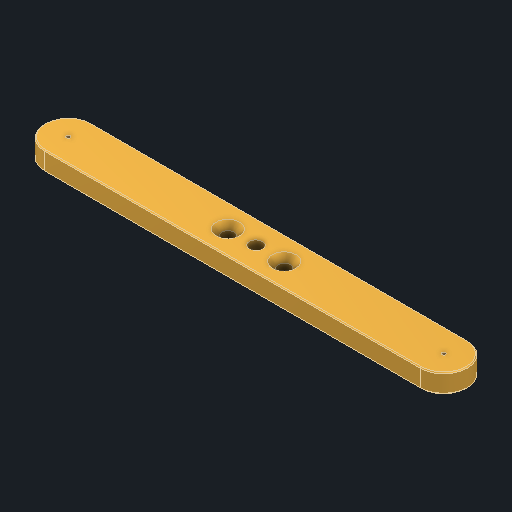
# Autodesk Inventor part: Brass Plate
Saved by Autodesk Inventor 2027.1 (Build 311270010, 270A)
## iProperties
Created: 2025-09-16
Part Number: Brass Plate
Material: Brass, Soft Yellow
Document SubType Name: Modeling
Designer: SD
Density: 8.47 g/cm^3
Appearance: Brass - Satin
Mass: 496.608 g
Surface Area: 177.89 cm^2
Volume: 58.6314 cm^3
Project: Automatic Tea Steeping mechanism
Length: 225.000 mm
Width: 25.000 mm
Thickness: 10.000 mm
BOM-Mass: 0.49661
BOM-Area: 0.018
Procurement: Fabricate - 1st round
Build Stage: 1
Preferred Material: C36000 Brass
Author: SD
Title: Brass Plate
Autodesk Inventor part; units mm, degrees
ref_plane "YZ Plane" through (0, 0, 0) normal (1, 0, 0) x (0, 1, 0)
ref_plane "XZ Plane" through (0, 0, 0) normal (0, 1, 0) x (-1, 0, 0)
ref_plane "XY Plane" through (0, 0, 0) normal (0, 0, 1) x (1, 0, 0)
sketch "Sketch1" plane through (0, 0, 0) normal (0, 1, 0) x (-1, 0, 0)
  line L0 (-112.5, 12.5) -> (112.5, 12.5)
  line L1 (112.5, 12.5) -> (112.5, -12.5)
  line L2 (112.5, -12.5) -> (-112.5, -12.5)
  line L3 (-112.5, -12.5) -> (-112.5, 12.5)
  line L4 (-112.5, 12.5) -> (112.5, -12.5) construction
  line L5 (112.5, 12.5) -> (-112.5, -12.5) construction
  point P0 (0, 0)
  dimension "Length" = 225
  dimension "Width" = 25
  constraints: 12 end point, 2 midpoint, 2 parallel, 1 horizontal, 1 perpendicular
  measures "Length" distance of L1.end L2.end
  measures "Width" distance of L0.end L1.end
extrude "Extrusion1" add sketch "Sketch1" along normal mid plane 10
sketch "Sketch2" plane through (0, 5, 0) normal (0, 1, 0) x (1, 0, 0)
  circle A0 centre (0, 0) radius 3.5
  dimension "d4" = 7
  constraints: 1 centre point, 1 coincident
  measures "d4" diameter of A0
extrude "Extrusion2" cut sketch "Sketch2" against normal up to surface (10 mm away)
sketch "Sketch3" plane through (0, 5, 0) normal (0, 1, 0) x (1, 0, 0)
  circle A0 centre (0, 0) radius 3.5 projected
  point P0 (-15, 0)
  point P1 (15, 0)
  dimension "d7" = 30
  dimension "d8" = 15
  constraints: 2 horizontal alignment
  measures "d7" distance of point (15, 0) point (-15, 0)
  measures "d8" distance of A0.centre point (15, 0)
hole "Hole1" at (-15, 5, 0) at (15, 5, 0) direction (0, -1, 0) diameter 6.5 end through all countersink diameter 12.6 countersink angle 90
sketch "Sketch4" plane through (0, 5, 0) normal (0, 1, 0) x (1, 0, 0)
  point P0 (0, 0)
  point P1 (-100, 0)
  point P2 (100, 0)
  dimension "d16" = 200
  dimension "d17" = 100
  constraints: 2 horizontal alignment
  measures "d16" distance of point (100, 0) point (-100, 0)
  measures "d17" distance of point (0, 0) point (100, 0)
hole "Hole2" at (-100, 5, 0) at (100, 5, 0) direction (0, -1, 0) diameter 2.1211 end through all thread size "M2.5x0.35" class "6H" standard "ISO Metric profile"
fillet "Fillet1" radius 12.5 4 edges at (112.5, 0, 12.5) (112.5, 0, -12.5) (-112.5, 0, 12.5) (-112.5, 0, -12.5)
chamfer "Chamfer1" distance 0.5 angle 45 16 edges at (0, 5, 12.5) (112.5, 5, 0) (108.8389, 5, 8.8389) (108.8389, 5, -8.8389) (0, 5, -12.5) (-108.8389, 5, 8.8389) (-108.8389, 5, -8.8389) (-112.5, 5, 0) (0, -5, 12.5) (-108.8389, -5, 8.8389) (-108.8389, -5, -8.8389) (-112.5, -5, 0) (0, -5, -12.5) (112.5, -5, 0) (108.8389, -5, 8.8389) (108.8389, -5, -8.8389)
equation "\"d8\" = 0.5 * d7"
equation "\"d17\" = 0.5 * d16"
body "Solid1"
